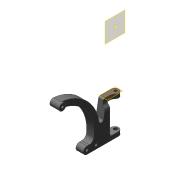
# Autodesk Inventor part: thumb_base
Saved by Autodesk Inventor 2014 (Build 180170000, 170)
## iProperties
Created: 2015-05-30
Part Number: thumb_base
Material: Generic
Document SubType Name: Modeling
Designer: Martin
Density: 1 g/cm^3
Appearance: Default
Author: Martin
Autodesk Inventor part; units mm, degrees
ref_plane "YZ Plane" through (0, 0, 0) normal (1, 0, 0) x (0, 1, 0)
ref_plane "XZ Plane" through (0, 0, 0) normal (0, 1, 0) x (-1, 0, 0)
ref_plane "plane_main" through (10, -20, 0) normal (1, 0, 0) x (0, 1, 0)
sketch "Sketch1" plane through (10, -20, 0) normal (1, 0, 0) x (0, 1, 0)
  line L0 (0, -108) -> (0, 18)
  line L1 (20, -86.5) -> (15.45, -86.5) projected
  line L2 (-1.875, -97.5779) -> (1.875, -97.5779) projected
  line L3 (-2.5, -65.2) -> (2.5, -65.2) projected
  line L4 (4, -96.0779) -> (-9.3, -96.0779)
  line L5 (-9.3, -96.0779) -> (-9.3, -64.7)
  line L6 (-9.3, -64.7) -> (4, -64.7)
  line L7 (4, -64.7) -> (4, -60.2)
  line L8 (4, -60.2) -> (-13.4946, -60.2)
  line L9 (-13.4946, -60.2) -> (-19.3, -92.5779)
  line L10 (-19.3, -92.5779) -> (-34.3, -92.5779)
  line L11 (-34.3, -92.5779) -> (-34.3, -100.5779) construction
  line L12 (-34.3, -100.5779) -> (4, -100.5779)
  line L13 (4, -96.0779) -> (4, -100.5779)
  line L14 (-7.3, -86.5) -> (-7.3, -65.2) projected
  arc A0 (-34.3, -92.5779) -> (-34.3, -100.5779) centre (-34.3, -96.5779) ccw
  circle A1 centre (-34.3, -96.5779) radius 1.25
  circle A2 centre (-24.3, -96.5779) radius 1.25
  line L15 (-34.3, -96.5779) -> (-24.3, -96.5779) construction
  point P0 (20, 0)
  dimension "d0" = 0.5
  dimension "d1" = 1.5
  dimension "d2" = 4.5
  dimension "d3" = 4.5
  dimension "d4" = 8
  dimension "d7" = 31.3779
  dimension "d8" = 2.5
  dimension "d9" = 10
  dimension "d10" = 15
  dimension "d11" = 10
  dimension "d12" = 2
  dimension "d21" = 4
  dimension "d22" = 4
  constraints: 24 end point, 7 perpendicular, 4 parallel, 3 centre point, 2 point on circle, 2 tangent, 1 coincident, 1 equal radius, 1 vertical, 2 other
  measures "d0" distance between parallel lines of L6 L3
  measures "d1" distance between parallel lines of L4 L2
  measures "d2" distance of L6.end L7.end
  measures "d3" distance between parallel lines of L4 L12
  measures "d4" distance between parallel lines of L12 L10
  measures "d7" distance of L4.end L5.end
  measures "d8" diameter of A1
  measures "d9" distance of L15.start L15.end
  measures "d10" horizontal distance of L9.end A0.centre
  measures "d11" horizontal distance of L4.end L9.end
  measures "d12" distance between parallel lines of L14 L5
  measures "d21" distance between parallel lines of L0 L7
  measures "d22" distance between parallel lines of L0 L13
extrude "ext_main" add sketch "Sketch1" along normal mid plane 8 contours L12 A0 L10 L9 L8 L0 L6 L5 L4 | L0 L4 L13 L12 | L0 L8 L7 L6
fillet "Fillet1" radius 2 3 edges at (10, -39.3, -92.5779) (10, -33.4946, -60.2) (10, -29.3, -96.0779)
sketch "Sketch3" plane through (6, -16, -60.2) normal (0, 0, 1) x (1, 0, 0)
  circle A0 centre (4, -3.2197) radius 1.5
  point P0 (-6, 16)
  dimension "d17" = 3
  constraints: 1 centre point, 1 coincident, 1 other
  measures "d17" diameter of A0
extrude "ext_cut_topbore" cut sketch "Sketch3" against normal up to surface (4.5 mm away)
fillet "Fillet2" radius 4 4 edges at (14, -16, -62.45) (6, -16, -62.45) (14, -16, -98.3279) (6, -16, -98.3279)
ref_plane "Work Plane2" through (6, -31.8213, -60.2) normal (0, 0, 1) x (1, 0, 0)
sketch "Sketch5" plane through (6, -31.8213, -60.2) normal (0, 0, 1) x (1, 0, 0)
  line L0 (8, 11.8213) -> (8, 0) projected
  circle A0 centre (14, 4.111) radius 9
  circle A1 centre (4, 12.6016) radius 1.5 projected
  arc A2 (8, 11.8213) -> (0, 11.8213) centre (4, 11.8213) ccw projected
  arc A3 (7.3667, 10.1937) -> (8, 11.8213) centre (5.5918, 11.8213) ccw
  line L1 (8, 11.8213) -> (8, 10.8192)
  line L2 (5, 4.111) -> (5, -4.889)
  line L3 (5, -4.889) -> (14, -4.889)
  point P0 (-6, 31.8213)
  point P1 (4, 12.611)
  dimension "d27" = 18
  dimension "d28" = 8.5
  dimension "d29" = 10
  constraints: 6 end point, 6 point on circle, 4 tangent, 2 centre point, 1 parallel, 1 perpendicular, 1 point on line, 1 other
  measures "d27" diameter of A0
  measures "d28" vertical distance of point (4, 12.611) A0.centre
  measures "d29" horizontal distance of point (4, 12.611) A0.centre
extrude "ext_cut_motor_cutway" cut sketch "Sketch5" along normal mid plane 15 contours L0 A0 A3 | A0 | A0 L3 L2
fillet "Fillet4" [suppressed]
sketch "Sketch6" plane through (10, -20, 0) normal (1, 0, 0) x (0, 1, 0)
  line L0 (0, -96.0779) -> (0, -96.0779) projected
  line L1 (-7.3, -96.0779) -> (0, -96.0779) projected
  line L2 (0, -96.0779) -> (-7.3, -96.0779) projected
  line L3 (0, -100.5779) -> (0, -100.5779) projected
  line L4 (-34.3, -100.5779) -> (0, -100.5779) projected
  line L5 (0, -100.5779) -> (-34.3, -100.5779) projected
  line L6 (0.7803, -108) -> (0.7803, 18) construction
  line L7 (0.7803, -96.0779) -> (0.7803, -100.5779)
  line L8 (1.5303, -100.5779) -> (1.5303, -98.2779)
  line L9 (1.5303, -98.2779) -> (2.7803, -98.2779)
  line L10 (2.7803, -98.2779) -> (2.7803, -96.0779)
  line L11 (2.7803, -96.0779) -> (0.7803, -96.0779)
  line L12 (0, -96.0779) -> (-7.3, -96.0779) projected
  line L13 (0.7803, -100.5779) -> (1.5303, -100.5779)
  line L14 (-34.3, -100.5779) -> (0, -100.5779) projected
  point P0 (20, 0)
  dimension "d37" = 0.75
  dimension "d38" = 2
  dimension "d39" = 2.2
  constraints: 14 end point, 4 parallel, 4 point on line, 1 perpendicular, 1 vertical, 2 other
  measures "d37" distance between parallel lines of L6 L8
  measures "d38" distance between parallel lines of L6 L10
  measures "d39" distance between parallel lines of L11 L9
revolve "revolution_servohubfit" cut sketch "Sketch6" angle 360 about axis through (10, -19.2197, -108) along (0, 0, 1)
sketch "Sketch7" plane through (10, -20, 0) normal (1, 0, 0) x (0, 1, 0)
  line L0 (0, -100.5779) -> (0, -96.0779) projected
  line L1 (0, -100.5779) -> (-34.3, -100.5779) projected
  arc A0 (-34.3, -92.5779) -> (-34.3, -100.5779) centre (-34.3, -96.5779) ccw projected
  line L2 (-34.3, -92.5779) -> (-20.9733, -92.5779) projected
  arc A1 (-20.9733, -92.5779) -> (-19.0047, -90.9309) centre (-20.9733, -90.5779) ccw projected
  line L3 (-19.0047, -90.9309) -> (-13.7899, -61.847) projected
  arc A2 (-11.8213, -60.2) -> (-13.7899, -61.847) centre (-11.8213, -62.2) ccw projected
  line L4 (-11.8213, -60.2) -> (0, -60.2) projected
  line L5 (0, -64.7) -> (0, -60.2) projected
  line L6 (0, -64.7) -> (-9.3, -64.7) projected
  line L7 (-9.3, -64.7) -> (-9.3, -94.0779) projected
  arc A3 (-9.3, -94.0779) -> (-7.3, -96.0779) centre (-7.3, -94.0779) ccw projected
  line L8 (-7.3, -96.0779) -> (0, -96.0779) projected
  circle A4 centre (-34.3, -96.5779) radius 1.25 projected
  circle A5 centre (-24.3, -96.5779) radius 1.25 projected
  line L9 (-34.3, -96.5779) -> (-24.3, -96.5779)
  line L10 (-24.3, -96.5779) -> (-24.3, -86.5779)
  line L11 (-24.3, -86.5779) -> (-62.8673, -40.6152) construction
  line L12 (-24.3, -86.5779) -> (-34.3, -96.5779) construction
  circle A6 centre (-62.8673, -40.6152) radius 1.25
  arc A7 (-24.3, -86.5779) -> (-62.8673, -40.6152) centre (-67.714, -83.8444) ccw construction
  line L13 (-34.3911, -55.8831) -> (-43.5836, -63.5965) construction
  circle A8 centre (-62.8673, -40.6152) radius 3.75
  line L14 (-19.0047, -90.9309) -> (-13.7899, -61.847) projected
  arc A9 (-24.3, -86.5779) -> (-59.1621, -41.1933) centre (-67.714, -83.8444) ccw
  arc A10 (-27.6511, -92.5779) -> (-60.4568, -43.4879) centre (-67.714, -83.8444) ccw
  line L15 (-19.2993, -92.5738) -> (-19.2993, -100.5779)
  line L16 (-24.3, -92.5779) -> (-24.3, -95.3279)
  line L17 (-19.2993, -95.3279) -> (-24.3, -95.3279)
  arc A11 (-21.0627, -76.3468) -> (-16.3973, -76.3889) centre (-18.7264, -75.9713) ccw
  line L18 (-14.8394, -67.7) -> (-19.0047, -90.9309) projected
  arc A12 (-62.0154, -36.9632) -> (-62.0154, -36.9632) centre (-74.2254, -89.308) ccw
  arc A13 (-21.2777, -92.5754) -> (-62.4494, -36.8886) centre (-67.714, -83.8444) ccw
  point P0 (20, 0)
  point P1 (-15.2647, -70.072)
  dimension "d41" = 60
  dimension "d43" = 10
  dimension "d44" = 140
  dimension "d45" = 2.5
  dimension "d46" = 12
  dimension "d53" = 2.5
  constraints: 19 point on circle, 16 end point, 8 centre point, 8 point on line, 4 perpendicular, 3 concentric, 3 tangent, 2 coincident, 2 midpoint, 1 horizontal, 1 line through centre, 1 parallel, 1 vertical alignment, 1 other
  measures "d41" distance of L10.end L11.end
  measures "d43" distance of L9.end L10.end
  measures "d44" angle of L10 L11
  measures "d45" diameter of A6
  measures "d46" distance of L13.start L13.end
  measures "d53" radial gap between concentric circles of A6 A8
extrude "Extrusion7" add sketch "Sketch7" along normal mid plane 8 contours A13 A12 | A12 A8 A13 | A12 A1 L2 L10 A9 A8 | A8 | A11 L3 A1 A12 A13 | A10 A8 A9 L10 L2
fillet "Fillet7" radius 5 2 edges at (10, -80.4568, -43.4879) (10, -47.6511, -92.5779)
sketch "Sketch11" plane through (6, -20, 0) normal (-1, 0, 0) x (0, 0, 1)
  circle A0 centre (-40.6152, -62.8673) radius 1.25 projected
  arc A1 (-44.1033, -61.4905) -> (-36.8886, -62.4494) centre (-40.6152, -62.8673) ccw projected
  line L0 (-96.0779, -7.3) -> (-96.0779, 0) projected
  circle A2 centre (-40.6152, -62.8673) radius 2
  line L1 (-42.6152, -62.8673) -> (-38.6152, -62.8673) construction
  line L2 (-120.6935, 20) -> (20.1156, 20) projected
  line L3 (-42.0435, -61.4673) -> (-39.1869, -61.4673)
  line L4 (-42.0435, -64.2673) -> (-39.1869, -64.2673)
  point P0 (0, 20)
  dimension "d68" = 4
  dimension "d69" = 2.8
  constraints: 6 end point, 6 point on circle, 3 parallel, 2 symmetric about line, 1 centre point, 1 coincident, 1 midpoint, 1 perpendicular
  measures "d68" diameter of A2
  measures "d69" distance between parallel lines of L4 L3
extrude "Extrusion11" cut sketch "Sketch11" against normal blind 5.75 contours A0 | A2 L4 L3
sketch "Sketch12" plane through (14, -20, 0) normal (1, 0, 0) x (0, 0, -1)
  circle A0 centre (40.6152, -62.8673) radius 1.25 projected
  arc A1 (36.8886, -62.4494) -> (44.1033, -61.4905) centre (40.6152, -62.8673) ccw projected
  circle A2 centre (40.6152, -62.8673) radius 3.75
  point P0 (0, 20)
  constraints: 1 centre point, 1 coincident, 1 concentric
extrude "Extrusion12" add sketch "Sketch12" along normal blind 2
sketch "Sketch15" plane through (6, -20, 0) normal (-1, 0, 0) x (0, 0, 1)
  arc A0 (-36.8886, -62.4494) -> (-76.3468, -21.0627) centre (-83.8444, -67.714) ccw projected
  arc A1 (-76.3889, -16.3973) -> (-76.3468, -21.0627) centre (-75.9713, -18.7264) ccw projected
  line L0 (-76.3889, -16.3973) -> (-61.847, -13.7899) projected
  arc A2 (-61.847, -13.7899) -> (-60.2, -11.8213) centre (-62.2, -11.8213) ccw projected
  line L1 (-60.2, -11.8213) -> (-60.2, 0) projected
  arc A3 (-60.2, -11.8213) -> (-50.8988, -33.8444) centre (-29.4767, -11.8213) ccw
  circle A4 centre (-75.9713, -18.7264) radius 2.3662
  line L2 (-76.3889, -16.3973) -> (-61.847, -13.7899)
  arc A5 (-61.847, -13.7899) -> (-60.2, -11.8213) centre (-62.2, -11.8213) ccw
  arc A6 (-50.8988, -33.8444) -> (-76.3468, -21.0627) centre (-83.8444, -67.714) ccw
  point P0 (0, 20)
  constraints: 9 tangent, 7 point on circle, 4 centre point, 2 end point, 1 coincident, 1 collinear, 1 concentric
extrude "Extrusion14" add sketch "Sketch15" against normal blind 8 contours A0 A4 L0 A2 A3
sketch "Sketch16" plane through (6, -31.8213, -60.2) normal (0, 0, 1) x (1, 0, 0)
  line L0 (8, -3.018) -> (5, -3.018) projected
  line L1 (8, 2.5213) -> (8, -3.018) projected
  line L2 (5, 2.5213) -> (8, 2.5213) projected
  line L3 (5, -3.018) -> (5, 2.5213) projected
  line L4 (8, 0) -> (8, -22.023) projected
  line L5 (5, -3.018) -> (5, -7.9972)
  arc A0 (5, -7.9972) -> (8, -13.6434) centre (11.8132, -7.9972) ccw
  line L6 (8, -13.6434) -> (8, -3.018)
  line L7 (8, -3.018) -> (5, -3.018)
  point P0 (-6, 31.8213)
  constraints: 6 end point, 2 point on circle, 1 centre point, 1 collinear, 1 parallel, 1 perpendicular, 1 point on line, 1 tangent
extrude "Extrusion15" cut sketch "Sketch16" against normal blind 7.5 and the other way blind 4
sketch "Sketch17" plane through (6, -31.8213, -67.7) normal (0, 0, 1) x (1, 0, 0)
  line L0 (8, 2.5213) -> (8, -13.6434) projected
  line L1 (5, 2.5213) -> (8, 2.5213) projected
  line L2 (5, 2.5213) -> (8, 1.1224)
  line L3 (8, 1.1224) -> (8, 2.5213)
  line L4 (8, 2.5213) -> (5, 2.5213)
  point P0 (-6, 31.8213)
  dimension "d85" = 25
  constraints: 6 end point, 2 perpendicular, 1 point on line
  measures "d85" angle of L4 L2
extrude "Extrusion16" cut sketch "Sketch17" against normal blind 25.25
equation "\"d8\" = screw_m2_bore_loose"
equation "\"d21\" = 0.5 * model_main_thickness"
equation "\"d22\" = 0.5 * model_main_thickness"
equation "\"d5\" = model_main_thickness"
equation "\"d17\" = screw_m3_bore_selfthreading"
equation "\"d20\" = 0.5 * model_main_thickness"
equation "\"d36\" = 0.5 * model_main_thickness"
equation "\"d37\" = 0.5 * model_servoscrew_diam"
equation "\"d38\" = 0.5 * model_servohub_diam"
equation "\"d45\" = screw_m2_bore_loose"
equation "\"d54\" = model_main_thickness"
equation "\"d76\" = model_main_thickness"
equation "\"model_main_thickness\" = 8"
equation "\"model_servoscrew_diam\" = 1.5"
equation "\"model_servohub_diam\" = 4"
equation "\"screw_m2_bore_loose\" = 2.5"
equation "\"screw_m3_bore_selfthreading\" = 3"
body "Solid1"
